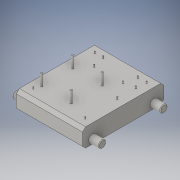
# Autodesk Inventor part: chassis
Saved by Autodesk Inventor 2016 (Build 200138000, 138)
## iProperties
Created: 2016-12-09
Part Number: chassis
Material: Generic
Document SubType Name: Modeling
Designer: lachesis
Density: 1 g/cm^3
Appearance: Default
Author: lachesis
Autodesk Inventor part; units mm, degrees
ref_plane "YZ Plane" through (0, 0, 0) normal (1, 0, 0) x (0, 1, 0)
ref_plane "XZ Plane" through (0, 0, 0) normal (0, 1, 0) x (-1, 0, 0)
ref_plane "XY Plane" through (0, 0, 0) normal (0, 0, 1) x (1, 0, 0)
sketch "Sketch1" plane through (0, 0, 0) normal (0, 1, 0) x (-1, 0, 0)
  line L0 (100.7745, 123.6) -> (-100.7745, 123.6)
  line L1 (-100.7745, 123.6) -> (-100.7745, -123.6)
  line L2 (-100.7745, -123.6) -> (100.7745, -123.6)
  line L3 (100.7745, -123.6) -> (100.7745, 123.6)
  point P0 (0, 0)
  point P1 (100.7745, 0)
  point P2 (0, 123.6)
  dimension "d0" = 247.2
  dimension "d1" = 201.549
  constraints: 8 end point, 2 midpoint, 2 parallel, 1 horizontal, 1 horizontal alignment, 1 perpendicular, 1 vertical alignment
  measures "d0" distance between parallel lines of L2 L0
  measures "d1" distance between parallel lines of L1 L3
extrude "Extrusion1" add sketch "Sketch1" along normal blind 56.4
sketch "Sketch3" plane through (100.7745, 0, 123.6) normal (1, 0, 0) x (0, 0, -1)
  circle A0 centre (30.111, 15.25) radius 11.25
  circle A1 centre (217.089, 15.25) radius 11.25
  line L0 (247.2, 0) -> (0, 0) projected
  line L1 (0, 0) -> (0, 56.4) projected
  line L2 (247.2, 56.4) -> (0, 56.4) projected
  line L3 (247.2, 0) -> (247.2, 56.4) projected
  point P0 (123.6, 0)
  dimension "d12" = 4
  dimension "d13" = 4
  dimension "d50" = 30.111
  dimension "d51" = 15.25
  dimension "d52" = 15.25
  dimension "d53" = 30.111
  constraints: 2 centre point
  measures "d12" distance edge to line of A0 L0
  measures "d13" distance edge to line of A1 L0
  measures "d50" distance from line of L1 A0.centre
  measures "d51" distance from line of A0.centre L0
  measures "d52" distance from line of L0 A1.centre
  measures "d53" distance from line of L3 A1.centre
extrude "Extrusion3" add sketch "Sketch3" along normal blind 30.94 contours A0 | A1
sketch "Sketch5" plane through (-100.7745, 0, -123.6) normal (-1, 0, 0) x (0, 0, 1)
  circle A0 centre (217.089, 15.25) radius 11.25 projected
  circle A1 centre (30.111, 15.25) radius 11.25 projected
  circle A2 centre (30.111, 15.25) radius 11.25
  circle A3 centre (217.089, 15.25) radius 11.25
  point P0 (123.6, 0)
  constraints: 2 centre point, 2 coincident, 2 concentric
extrude "Extrusion5" add sketch "Sketch5" along normal blind 30.94
sketch "Sketch8" plane through (100.7745, 0, 123.6) normal (1, 0, 0) x (0, 0, -1)
  line L0 (0, 0) -> (0, 56.4) projected
  line L1 (0, 47.0005) -> (9.3472, 56.4)
  line L2 (0, 9.3995) -> (9.3472, 0)
  line L3 (0, 56.4) -> (247.2, 56.4) projected
  line L4 (237.8528, 56.4) -> (247.2, 47.0005)
  line L5 (247.2, 0) -> (247.2, 56.4) projected
  line L6 (247.2, 9.3995) -> (237.8528, 0)
  line L7 (0, 0) -> (247.2, 0) projected
  point P0 (123.6, 0)
  dimension "d22" = 13.256
  dimension "d23" = 135.16
  dimension "d24" = 135.16
  dimension "d25" = 135.16
  dimension "d26" = 135.16
  constraints: 8 end point, 8 point on line, 3 equal length
  measures "d22" distance of L1.start L1.end
  measures "d23" angle of L0 L1
  measures "d24" angle of L0 L2
  measures "d25" angle of L5 L6
  measures "d26" angle of L5 L4
extrude "Extrusion6" cut sketch "Sketch8" against normal through all contours L0 L2 L7 | L0 L3 L1 | L6 L5 L7 | L3 L5 L4
sketch "Sketch9" plane through (0, 56.4, 0) normal (0, 1, 0) x (1, 0, 0)
  circle A0 centre (78.9745, -93.586) radius 1.651
  line L0 (100.7745, -123.6) -> (-100.7745, -123.6) projected
  line L1 (100.7745, -114.2528) -> (100.7745, 114.2528) projected
  circle A1 centre (78.9745, 93.586) radius 1.651
  circle A2 centre (-78.9745, 93.586) radius 1.651
  circle A3 centre (-78.9745, -93.586) radius 1.651
  line L2 (-100.7745, 123.6) -> (100.7745, 123.6) projected
  line L3 (-100.7745, 114.2528) -> (-100.7745, -114.2528) projected
  point P0 (0, 0)
  dimension "d29" = 30.014
  dimension "d30" = 21.8
  dimension "d31" = 3.302
  dimension "d32" = 3.302
  dimension "d33" = 3.302
  dimension "d34" = 3.302
  dimension "d35" = 21.8
  dimension "d36" = 30.014
  dimension "d37" = 21.8
  dimension "d38" = 30.014
  dimension "d39" = 21.8
  dimension "d40" = 30.014
  constraints: 4 centre point
  measures "d29" distance from line of A0.centre L0
  measures "d30" distance from line of A0.centre L1
  measures "d31" diameter of A0
  measures "d32" diameter of A1
  measures "d33" diameter of A2
  measures "d34" diameter of A3
  measures "d35" distance from line of L1 A1.centre
  measures "d36" distance from line of L2 A1.centre
  measures "d37" distance from line of L3 A2.centre
  measures "d38" distance from line of L2 A2.centre
  measures "d39" distance from line of L3 A3.centre
  measures "d40" distance from line of L0 A3.centre
extrude "Extrusion7" add sketch "Sketch9" along normal blind 4.763
sketch "Sketch10" plane through (0, 56.4, 0) normal (0, 1, 0) x (1, 0, 0)
  circle A0 centre (76.4345, 63.106) radius 1.905
  circle A1 centre (76.4345, 6.591) radius 1.905
  line L0 (100.7745, -114.2528) -> (100.7745, 114.2528) projected
  line L1 (-100.7745, 123.6) -> (100.7745, 123.6) projected
  point P0 (0, 0)
  dimension "d43" = 24.34
  dimension "d44" = 3.81
  dimension "d45" = 3.81
  dimension "d46" = 60.494
  dimension "d47" = 56.515
  constraints: 2 centre point, 1 vertical alignment
  measures "d43" distance from line of L0 A0.centre
  measures "d44" diameter of A0
  measures "d45" diameter of A1
  measures "d46" distance from line of A0.centre L1
  measures "d47" distance of A1.centre A0.centre
extrude "Extrusion8" add sketch "Sketch10" along normal blind 6.35
fillet "Fillet1" radius 2 4 edges at (131.7145, 15.25, 104.739) (131.7145, 15.25, -82.239) (-131.7145, 15.25, -104.739) (-131.7145, 15.25, 82.239)
sketch "Sketch11" plane through (0, 56.4, 0) normal (0, 1, 0) x (1, 0, 0)
  circle A0 centre (76.4345, 63.106) radius 1.905 projected
  circle A1 centre (76.4345, 6.591) radius 1.905 projected
  circle A2 centre (-78.9745, 93.586) radius 1.651 projected
  circle A3 centre (78.9745, -93.586) radius 1.651 projected
  circle A4 centre (78.9745, 93.586) radius 1.651 projected
  circle A5 centre (-78.9745, -93.586) radius 1.651 projected
  line L0 (100.7745, 114.2528) -> (-100.7745, 114.2528) projected
  line L1 (-100.7745, 114.2528) -> (-100.7745, -114.2528) projected
  line L2 (-100.7745, -114.2528) -> (100.7745, -114.2528) projected
  line L3 (100.7745, -114.2528) -> (100.7745, 114.2528) projected
  circle A6 centre (-43.9615, 56.5758) radius 1.651
  circle A7 centre (-52.8515, 92.6438) radius 1.651
  circle A8 centre (52.8815, 92.6438) radius 1.651
  circle A9 centre (43.9915, 56.5758) radius 1.651
  point P0 (0, 0)
  dimension "d58" = 21.609
  dimension "d62" = 21.609
  dimension "d63" = 3.302
  dimension "d79" = 87.953
  dimension "d80" = 105.733
  dimension "d81" = 36.068
  dimension "d82" = 36.068
  dimension "d83" = 47.893
  dimension "d84" = 56.783
  constraints: 4 centre point, 3 equal radius
  measures "d58" distance from line of A7.centre L0
  measures "d62" distance from line of L0 A8.centre
  measures "d63" diameter of A6
  measures "d79" distance of A9.centre A6.centre
  measures "d80" distance of A8.centre A7.centre
  measures "d81" vertical distance of A6.centre A7.centre
  measures "d82" vertical distance of A9.centre A8.centre
  measures "d83" distance from line of A8.centre L3
  measures "d84" distance from line of A9.centre L3
extrude "Extrusion9" add sketch "Sketch11" along normal blind 6.35 contours A6 | A7 | A8 | A9
sketch "Sketch12" plane through (0, 56.4, 0) normal (0, 1, 0) x (1, 0, 0)
  circle A0 centre (52.8815, 92.6438) radius 1.651 projected
  circle A1 centre (-43.9615, 56.5758) radius 1.651 projected
  circle A2 centre (-52.8515, 92.6438) radius 1.651 projected
  circle A3 centre (43.9915, 56.5758) radius 1.651 projected
  circle A4 centre (76.4345, 63.106) radius 1.905 projected
  circle A5 centre (76.4345, 6.591) radius 1.905 projected
  circle A6 centre (-78.9745, 93.586) radius 1.651 projected
  circle A7 centre (78.9745, -93.586) radius 1.651 projected
  circle A8 centre (78.9745, 93.586) radius 1.651 projected
  circle A9 centre (-78.9745, -93.586) radius 1.651 projected
  line L0 (100.7745, 114.2528) -> (-100.7745, 114.2528) projected
  line L1 (-100.7745, 114.2528) -> (-100.7745, -114.2528) projected
  line L2 (-100.7745, -114.2528) -> (100.7745, -114.2528) projected
  line L3 (100.7745, -114.2528) -> (100.7745, 114.2528) projected
  circle A10 centre (-72.8345, 20.3292) radius 2.9845
  circle A11 centre (17.0815, 20.3292) radius 2.9845
  circle A12 centre (17.0815, -74.1588) radius 2.9845
  circle A13 centre (-72.8345, -74.1588) radius 2.9845
  point P0 (0, 0)
  dimension "d66" = 27.94
  dimension "d67" = 27.94
  dimension "d68" = 117.856
  dimension "d69" = 117.856
  dimension "d70" = 40.094
  dimension "d71" = 40.094
  dimension "d74" = 5.969
  dimension "d77" = 94.488
  dimension "d78" = 94.488
  constraints: 4 centre point, 3 equal radius
  measures "d66" distance from line of A10.centre L1
  measures "d67" distance from line of A13.centre L1
  measures "d68" distance from line of A11.centre L1
  measures "d69" distance from line of A12.centre L1
  measures "d70" distance from line of A13.centre L2
  measures "d71" distance from line of A12.centre L2
  measures "d74" diameter of A10
  measures "d77" distance of A10.centre A13.centre
  measures "d78" distance of A12.centre A11.centre
extrude "Extrusion10" add sketch "Sketch12" along normal blind 34.922 contours A10 | A11 | A12 | A13
equation "\"d13\" = d12"
equation "\"d52\" = d51"
equation "\"d53\" = d50"
equation "\"d24\" = d23"
equation "\"d25\" = d23"
equation "\"d26\" = d23"
equation "\"d32\" = d31"
equation "\"d33\" = d31"
equation "\"d34\" = d31"
equation "\"d35\" = d30"
equation "\"d36\" = d29"
equation "\"d37\" = d30"
equation "\"d38\" = d29"
equation "\"d39\" = d30"
equation "\"d40\" = d29"
equation "\"d45\" = d44"
equation "\"d62\" = d58"
equation "\"d82\" = d81"
equation "\"d67\" = d66"
equation "\"d69\" = d68"
equation "\"d71\" = d70"
equation "\"d78\" = d77"
body "Solid1"
